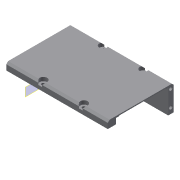
# Autodesk Inventor part: 01_Camera_Module_v0
Saved by Autodesk Inventor 2019 (Build 230136000, 136)
## iProperties
Created: 2021-09-09
Part Number: 01_Camera_Module_v0
Material: Generisch
Document SubType Name: Modeling
Designer: Muriel
Density: 1 g/cm^3
Appearance: Vorgabe
Author: Muriel
Autodesk Inventor part; units mm, degrees
ref_plane "Arbeitsebene6" through (-11.8704, 3.6846, 3.3435) normal (-1, 0, 0) x (0, 1, 0)
sketch "Skizze6" plane through (-11.8704, 3.6846, 3.3435) normal (-1, 0, 0) x (0, 1, 0)
  line L0 (7, 24) -> (7, 1) construction
  line L1 (7, 1) -> (8.5, 1) construction
  line L2 (8.5, 4) -> (8.5, 1) construction
  line L3 (8.5, 4) -> (11.3, 4) construction
  line L4 (11.3, 21) -> (11.3, 4) construction
  line L5 (8.5, 21) -> (11.3, 21) construction
  line L6 (8.5, 24) -> (8.5, 21) construction
  line L7 (7, 24) -> (8.5, 24) construction
  line L8 (8.5, -1) -> (8.5, 1) construction
  line L9 (7, -1) -> (8.5, -1) construction
  line L10 (7, -1) -> (7, 1) construction
  line L11 (8.5, 24) -> (8.5, 26) construction
  line L12 (7, 26) -> (8.5, 26) construction
  line L13 (7, 24) -> (7, 26) construction
  line L14 (12, -6.4) -> (8.1, -6.4)
  line L15 (3.3, 29.4) -> (12, 29.4)
  line L16 (12, 29.4) -> (12, -6.4)
  circle A0 centre (3.1, 20.5) radius 4 construction
  line L17 (7.6, 16) -> (7.6, 25) construction
  line L18 (7.6, 25) -> (-1.4, 25) construction
  line L19 (-1.4, 25) -> (-1.4, 16) construction
  line L20 (-1.4, 16) -> (7.6, 16) construction
  line L21 (3.3, 29.4) -> (-1.9, 29.4)
  line L22 (-1.9, 29.4) -> (-1.9, 11.5)
  line L23 (-1.9, 11.5) -> (8.1, 11.5)
  line L24 (3, 15.9) -> (3, 25.1)
  line L25 (5, 4.25) -> (5, 20.75) projected
  line L26 (11.3, 21) -> (11.3, 4) construction
  line L27 (7.7, 15.9) -> (7.7, 25.1)
  line L28 (7.7, 25.1) -> (-1.5, 25.1)
  line L29 (-1.5, 25.1) -> (-1.5, 15.9)
  line L30 (-1.5, 15.9) -> (7.7, 15.9)
  line L31 (3, 15.9) -> (3, 25.1)
  circle A1 centre (3.1, 20.5) radius 4 construction
  line L32 (7.6, 16) -> (7.6, 25) construction
  line L33 (7.6, 25) -> (-1.4, 25) construction
  line L34 (-1.4, 25) -> (-1.4, 16) construction
  line L35 (-1.4, 16) -> (7.6, 16) construction
  line L36 (-0.7, -1.5) -> (8.3, -1.5) construction
  line L37 (8.5, 7.7) -> (4.1628, 7.7) construction
  line L38 (-0.9, 7.7) -> (-0.9, -1.7) construction
  line L39 (8.1, -6.4) -> (8.1, 3.997) construction
  line L40 (8.1, -6.4) -> (8.1, 11.5)
  line L41 (4.1664, 7.9123) -> (4.1628, 7.7)
  point P0 (3, 11.5)
  dimension "d41" = 13.9
  dimension "d42" = 0.1
  dimension "d48" = 4.3
  dimension "d50" = 9
  dimension "d52" = 17.9
  dimension "d53" = 3.9
  dimension "d54" = 8.9
  dimension "d55" = 17.9
  dimension "d58" = 8.9
  constraints: 36 end point, 4 horizontal, 4 parallel, 4 point on line, 2 perpendicular, 2 vertical, 8 other
  measures "d41" distance between parallel lines of L22 L16
  measures "d42" distance between parallel lines of L20 L30
  measures "d48" distance between parallel lines of L28 L21
  measures "d50" distance from line of L23 A0.centre
  measures "d52" distance between parallel lines of L23 L21
  measures "d53" distance between parallel lines of L16 L40
  measures "d54" distance from line of L21 A1.centre
  measures "d55" distance between parallel lines of L14 L23
  measures "d58" distance from line of L16 A0.centre
ref_plane "Arbeitsebene7" through (-14.9704, 2.9846, -22.1565) normal (-1, 0, 0) x (0, 0, 1)
extrude "Extrusion6" add sketch "Skizze6" along normal up to surface (3.1 mm away)
sketch "Skizze7" plane through (-14.9704, 1.7846, -26.0565) normal (-1, 0, 0) x (0, 0, 1)
  line L0 (4.3, 0.4) -> (13.5, 0.4) projected
  line L1 (4.3, 9.6) -> (4.3, 0.4) projected
  line L2 (13.5, 9.6) -> (4.3, 9.6) projected
  line L3 (13.5, 0.4) -> (13.5, 9.6) projected
  line L4 (35.8, 10) -> (17.9, 10) projected
  line L5 (35.8, 13.9) -> (35.8, 10) projected
  line L6 (0, 13.9) -> (35.8, 13.9) projected
  line L7 (0, 0) -> (0, 13.9) projected
  line L8 (17.9, 0) -> (0, 0) projected
  line L9 (17.9, 10) -> (17.9, 0) projected
  circle A0 centre (8.9, 5) radius 4 construction
  circle A1 centre (8.9, 5) radius 4.2
  point P0 (26.0565, -1.7846)
  dimension "d141" = 8.4
  constraints: 1 centre point, 1 coincident
  measures "d141" diameter of A1
extrude "Extrusion7" add sketch "Skizze7" along normal blind 2 contours L1 L2 L3 L0 | L4 L9 L8 L7 L6 L5
ref_plane "Arbeitsebene8" through (34.8296, 10.6846, -20.6565) normal (1, 0, 0) x (0, 1, 0)
sketch "Skizze8" plane through (-11.8704, 3.6846, 3.3435) normal (1, 0, 0) x (0, 0, -1)
  line L0 (1, 7) -> (24, 7) construction
  line L1 (24, 7) -> (24, 8.5) construction
  line L2 (16.25, 8.5) -> (24, 8.5) construction
  line L3 (8.75, 8.5) -> (16.25, 8.5) construction
  line L4 (1, 8.5) -> (8.75, 8.5) construction
  line L5 (1, 7) -> (1, 8.5) construction
  line L6 (26, 8.5) -> (24, 8.5) construction
  line L7 (26, 7) -> (26, 8.5) construction
  line L8 (26, 7) -> (24, 7) construction
  line L9 (1, 8.5) -> (-1, 8.5) construction
  line L10 (-1, 7) -> (-1, 8.5) construction
  line L11 (1, 7) -> (-1, 7) construction
  line L12 (-6.4, 12) -> (-6.4, 8.1) construction
  line L13 (-6.4, 8.1) -> (11.5, 8.1) construction
  line L14 (11.5, 8.1) -> (11.5, -1.9) construction
  line L15 (11.5, -1.9) -> (29.4, -1.9) construction
  line L16 (29.4, -1.9) -> (29.4, 12) construction
  line L17 (29.4, 12) -> (-6.4, 12) construction
  line L18 (25.1, 7.7) -> (25.1, -1.5) construction
  line L19 (25.1, -1.5) -> (15.9, -1.5) construction
  line L20 (15.9, -1.5) -> (15.9, 7.7) construction
  line L21 (15.9, 7.7) -> (25.1, 7.7) construction
  line L22 (29.4, 12) -> (29.4, -1.9) projected
  line L23 (29.4, 12) -> (-6.4, 12) projected
  line L24 (29.4, -1.9) -> (26.4, -1.9)
  line L25 (26.4, -1.9) -> (26.4, 12)
  line L26 (26.4, 12) -> (29.4, 12)
  line L27 (29.4, 12) -> (29.4, -1.9)
  line L28 (26.4, 12) -> (25.1772, 12)
  line L29 (25.1772, 12) -> (25.1772, 9)
  line L30 (25.1772, 9) -> (26.4, 9)
  line L31 (26.4, 9) -> (26.4, 12)
  line L32 (-6.4, 12) -> (-6.4, 8.1) projected
  line L33 (-6.4, 8.1) -> (11.5, 8.1) projected
  line L34 (-6.4, 12) -> (-2, 12)
  line L35 (-2, 12) -> (-2, 8.1)
  line L36 (-2, 8.1) -> (-6.4, 8.1)
  line L37 (-6.4, 8.1) -> (-6.4, 12)
  line L38 (25.1772, 12) -> (-2, 12)
  line L39 (-2, 12) -> (-2, 12)
  line L40 (25.1772, 11.6) -> (25.1772, 12)
  line L41 (-0.2145, 9) -> (-2, 9)
  line L42 (-2, 9) -> (-2, 12)
  line L43 (-2, 12) -> (-0.2145, 12)
  line L44 (-0.2145, 12) -> (-0.2145, 9)
  line L45 (21, 8.5) -> (4, 8.5) construction
  line L46 (21, 8.5) -> (21, 11.3) construction
  line L47 (4, 11.3) -> (21, 11.3) construction
  line L48 (4, 8.5) -> (4, 11.3) construction
  line L49 (1, 7) -> (-1, 7) construction
  line L50 (29.4, 12) -> (26.4, 12)
  line L51 (26.4, 12) -> (26.4, -1.9)
  line L52 (26.4, -1.9) -> (29.4, -1.9)
  line L53 (29.4, -1.9) -> (29.4, 12)
  line L54 (1, 7) -> (-1, 7) projected
  line L55 (1, 8.5) -> (-1, 8.5) projected
  line L56 (1, 7) -> (24, 7) projected
  line L57 (24, 7) -> (24, 8.5) projected
  line L58 (16.25, 8.5) -> (24, 8.5) projected
  line L59 (8.75, 8.5) -> (16.25, 8.5) projected
  line L60 (1, 8.5) -> (8.75, 8.5) projected
  line L61 (1, 7) -> (1, 8.5) projected
  line L62 (1, 8.5) -> (-1, 8.5) projected
  line L63 (1, 7) -> (-1, 7) projected
  line L64 (1, 7) -> (1, 8.5) projected
  line L65 (-1, 7) -> (-1, 8.5) projected
  line L66 (25.1, -1.5) -> (15.9, -1.5) construction
  line L67 (1, 7) -> (-1, 7) construction
  line L68 (1, 7) -> (-1, 7) construction
  line L69 (-1, 7) -> (-1, 8.5) projected
  line L70 (26.4, -1.9) -> (24.9905, -1.9)
  line L71 (24.9905, -1.9) -> (24.9905, -0.65)
  line L72 (24.9905, -0.65) -> (26.4, -0.65)
  line L73 (26.4, -0.65) -> (26.4, -1.9)
  line L74 (26.4, -0.65) -> (23.4, -0.65)
  line L75 (23.4, -0.65) -> (23.4, 0.1)
  line L76 (23.4, 0.1) -> (26.4, 0.1)
  line L77 (26.4, 0.1) -> (26.4, -0.65)
  line L78 (26.4, 6.5844) -> (25.1772, 6.5844)
  line L79 (25.1772, 6.5844) -> (25.1772, 5.8344)
  line L80 (25.1772, 5.8344) -> (26.4, 5.8344)
  line L81 (26.4, 5.8344) -> (26.4, 6.5844)
  line L82 (-0.2145, 12) -> (25.1772, 12)
  line L83 (25.1772, 12) -> (25.1772, 11.4)
  line L84 (25.1772, 11.4) -> (-0.2145, 11.4)
  line L85 (-0.2145, 11.4) -> (-0.2145, 12)
  point P0 (3.3435, -3.6846)
  point P1 (23, -0.4)
  dimension "d60" = 1
  dimension "d61" = 0.5
  dimension "d63" = 0.5
  dimension "d65" = 0.4
  dimension "d133" = 3
  dimension "d134" = 0.75
  dimension "d135" = 0.75
  dimension "d136" = 0.6
  constraints: 78 end point, 19 parallel, 10 horizontal, 10 perpendicular, 6 point on line, 1 other
  measures "d60" distance between parallel lines of L10 L42
  measures "d61" distance from line of L41 L4.start
  measures "d63" distance between parallel lines of L6 L30
  measures "d65" distance between parallel lines of L25 L7
  measures "d133" distance of L75.end L76.end
  measures "d134" distance of L74.end L75.end
  measures "d135" distance of L79.end L78.end
  measures "d136" distance of L82.end L83.end
extrude "Extrusion8" add sketch "Skizze8" along normal blind 50 contours L22 L24 L25 L23 | L25 L30 L29 L23 | L70 L71 L72 L25 | L29 L84 L44 L23 | L72 L74 L75 L76 L25 | L44 L41 L35 L23 | L25 L80 L79 L78 | L35 L33 L32 L23
sketch "Skizze9" plane through (-16.9704, 15.6846, 9.7435) normal (0, 1, 0) x (1, 0, 0)
  line L0 (55.1, 0) -> (0, 0) projected
  line L1 (0, 35.8) -> (55.1, 35.8) projected
  line L2 (5.1, 7.9) -> (55.1, 7.9) projected
  line L3 (5.1, 3.5) -> (51.8, 3.5)
  line L4 (5.1, 4.4) -> (55.1, 4.4) projected
  line L5 (5.1, 32.8) -> (55.1, 32.8) projected
  line L6 (50.05, 34.05) -> (50.05, 1.75) construction
  line L7 (50.05, 1.75) -> (1.75, 1.75) construction
  line L8 (1.75, 1.75) -> (1.75, 34.05) construction
  line L9 (1.75, 34.05) -> (50.05, 34.05) construction
  line L10 (55.1, 35.8) -> (55.1, 0) projected
  circle A0 centre (40.4228, 1.75) radius 0.9758
  circle A1 centre (18.4228, 1.75) radius 1.1468
  line L11 (0, 0) -> (0, 35.8) projected
  point P0 (16.9704, 9.7435)
  point P1 (51.8, 7.9)
  point P2 (51.8, 3.9)
  point P3 (51.8, 32.3)
  point P4 (7.4228, 34.05)
  point P5 (18.4228, 34.05)
  point P6 (29.4228, 34.05)
  point P7 (40.4228, 34.05)
  point P8 (55.1, 4.4)
  point P9 (55.1, 32.8)
  dimension "d74" = 1.75
  dimension "d75" = 11
  dimension "d76" = 11
  dimension "d77" = 11
  dimension "d140" = 1.75
  constraints: 10 end point, 6 point on line, 2 centre point, 1 horizontal, 4 other
  measures "d74" distance between parallel lines of L1 L9
  measures "d75" distance of point (18.423, 34.05) point (7.423, 34.05)
  measures "d76" distance of point (29.423, 34.05) point (18.423, 34.05)
  measures "d77" distance of point (40.423, 34.05) point (29.423, 34.05)
  measures "d140" distance from line of A1.centre L0
hole "Bohrung1" at (23.4524, 15.6846, -24.3065) at (23.4524, 15.6846, 7.9935) at (1.4524, 15.6846, 7.9935) at (1.4524, 15.6846, -24.3065) direction (0, -1, 0) diameter 1.8 end through all counterbore diameter 4 counterbore depth 2
chamfer "Fase1" distance 1 angle 45 6 edges at (31.2751, 15.6846, -26.0565) (-8.2431, 15.6846, -26.0565) (12.4524, 15.6846, -26.0565) (12.4524, 15.6846, 9.7435) (-8.2431, 15.6846, 9.7435) (31.2751, 15.6846, 9.7435)
chamfer "Fase2" distance 1 angle 45 1 edges at (-11.8704, 6.7846, -12.5565)
sketch "Skizze11" plane through (34.8296, 1.9846, -26.0565) normal (0, 0, -1) x (-1, 0, 0)
  line L0 (49.8, 0.2) -> (49.8, 9.4) projected
  line L1 (47.7, 0.2) -> (47.7, 9.4) projected
  circle A0 centre (47.7, 4.8) radius 1.4
  point P0 (34.8296, -1.9846)
  dimension "d93" = 2.8
  constraints: 1 centre point, 1 midpoint
  measures "d93" diameter of A0
extrude "Extrusion10" cut sketch "Skizze11" against normal blind 10
sketch "Skizze12" plane through (-16.9704, 1.7846, -8.1565) normal (0, -1, 0) x (1, 0, 0)
  line L0 (5.1, -12.9) -> (55.1, -12.9) projected
  line L1 (5.1, -14.9) -> (55.1, -14.9) projected
  line L2 (5.1, -12.9) -> (55.1, -12.9) projected
  line L3 (5.1, -14.9) -> (5.1, -13.6) projected
  line L4 (5.1, -14.9) -> (55.1, -14.9) projected
  line L5 (55.1, -12.9) -> (55.1, -14.9) projected
  line L6 (55.1, -14.9) -> (41.1, -14.9)
  line L7 (41.1, -14.9) -> (41.1, -8.3617)
  line L8 (41.1, -8.3617) -> (55.1, -8.3617)
  line L9 (55.1, -8.3617) -> (55.1, -14.9)
  line L10 (5.1, -13.6772) -> (55.1, -13.6772) projected
  line L11 (5.1, -25.06) -> (5.1, 25.06) projected
  line L12 (5.1, -14.9) -> (21.1, -14.9)
  line L13 (21.1, -14.9) -> (21.1, -8.3617)
  line L14 (21.1, -8.3617) -> (5.1, -8.3617)
  line L15 (5.1, -8.3617) -> (5.1, -14.9)
  line L16 (5.1, -12.9) -> (5.1, -13.6) projected
  point P0 (16.9704, 8.1565)
  point P1 (51.8, -13.4)
  point P2 (51.8, -14.4)
  point P3 (5.1, -13.9)
  point P4 (5.1, -13.9)
  dimension "d113" = 36
  dimension "d132" = 0
  constraints: 16 end point, 4 parallel, 2 horizontal, 2 perpendicular, 1 point on line, 2 other
  measures "d113" distance between parallel lines of L7 L11
  measures "d132" distance from line of point (5.1, -14.9) L15
ref_plane "Arbeitsebene9" through (-11.8704, 12.1846, -22.6565) normal (0, 1, 0) x (0, 0, 1)
extrude "Extrusion11" cut sketch "Skizze12" against normal blind 13 contours L11 L14 L13 L0 | L0 L13 L10 L3 L11 | L7 L8 L9 L0 | L0 L5 L10 L7 | L13 L1 L3 L10 | L10 L5 L1 L7
sketch "Skizze13" plane through (38.1296, 10.1846, -23.0565) normal (1, 0, 0) x (0, 0, -1)
  line L0 (-32.3, 4.7) -> (-31.3, 5.7) projected
  line L1 (-32.3, 1.8) -> (-32.3, 4.7) projected
  line L2 (-28.4, 1.8) -> (-32.3, 1.8) projected
  line L3 (-28.4, 2.2) -> (-28.4, 1.8) projected
  line L4 (-24.4, 2.2) -> (-28.4, 2.2) projected
  line L5 (-24.4, 4.1) -> (-24.4, 2.2) projected
  line L6 (-4, 5.1) -> (-23.4, 5.1) projected
  line L7 (-3, 2.5) -> (-3, 4.1) projected
  line L8 (0, 2.5) -> (-3, 2.5) projected
  line L9 (0, 0) -> (0, 2.5) projected
  line L10 (-1, 0) -> (0, 0) projected
  line L11 (-1, -2) -> (-1, 0) projected
  line L12 (0, -4.4) -> (0, -3) projected
  line L13 (-1, -6.4) -> (-1, -5.4) projected
  line L14 (0, -6.4) -> (-1, -6.4) projected
  line L15 (0, -8.2) -> (0, -6.4) projected
  line L16 (3.5, -8.2) -> (0, -8.2) projected
  line L17 (3.5, 4.7) -> (3.5, -8.2) projected
  line L18 (2.5, 5.7) -> (3.5, 4.7) projected
  line L19 (-31.3, 5.7) -> (2.5, 5.7) projected
  circle A0 centre (1.4, -5.4) radius 0.9
  circle A1 centre (1.4, 3.4) radius 0.9
  line L20 (-23.4, 5.1) -> (-24.4, 4.1) projected
  line L21 (-3, 4.1) -> (-4, 5.1) projected
  line L22 (0, -3) -> (-1, -2) projected
  line L23 (-1, -5.4) -> (0, -4.4) projected
  point P0 (-23.0565, -10.1846)
  dimension "d101" = 1.8
  dimension "d102" = 1.8
  constraints: 2 centre point
  measures "d101" diameter of A0
  measures "d102" diameter of A1
extrude "Extrusion12" cut sketch "Skizze13" against normal blind 8 contours A0 | A1
sketch "Skizze15" plane through (-16.9704, 11.7846, -8.1565) normal (0, -1, 0) x (1, 0, 0)
  line L0 (5.1, 0) -> (0, 0) projected
  line L1 (5.1, 13.5) -> (5.1, 0) projected
  line L2 (0, 17.9) -> (55.1, 17.9) projected
  line L3 (13.1, 13.5131) -> (21.1, 13.5131)
  line L4 (21.1, 13.5131) -> (21.1, 8.0131)
  line L5 (21.1, 8.0131) -> (13.1, 8.0131)
  line L6 (13.1, 8.0131) -> (13.1, 13.5131)
  line L7 (41.1, -14.9) -> (41.1, -13.6772) projected
  line L8 (5.1, 13.5) -> (55.1, 13.5) projected
  line L9 (55.1, 84.35) -> (55.1, 11.7145) projected
  line L10 (41.1, 13.5) -> (55.1, 13.5)
  line L11 (55.1, 13.5) -> (55.1, 8)
  line L12 (55.1, 8) -> (41.1, 8)
  line L13 (41.1, 8) -> (41.1, 13.5)
  line L14 (41.1, -14.9) -> (55.1, -14.9)
  line L15 (55.1, -14.9) -> (55.1, -9.4)
  line L16 (55.1, -9.4) -> (41.1, -9.4)
  line L17 (41.1, -9.4) -> (41.1, -14.9)
  line L18 (5.1, 13.5) -> (55.1, 13.5) projected
  line L19 (55.1, 17.9) -> (55.1, 13.5) projected
  line L20 (0, 0) -> (0, 17.9) projected
  point P0 (16.9704, 8.1565)
  point P1 (134.9, 84.35)
  dimension "d116" = 8
  dimension "d117" = 8
  dimension "d120" = 5.5
  dimension "d122" = 5.5
  constraints: 24 end point, 6 parallel, 3 horizontal, 3 perpendicular, 2 point on line, 2 other
  measures "d116" distance of L4.end L5.end
  measures "d117" distance between parallel lines of L6 L1
  measures "d120" distance between parallel lines of L5 L3
  measures "d122" distance between parallel lines of L14 L16
extrude "Extrusion14" cut sketch "Skizze15" against normal blind 3 contours L8 L4 L5 L6 | L6 L3 L4 L8 | L9 L11 L12 L13 L8 | L7 L17 L16 L15 L14
chamfer "Fase4" distance 3 angle 45 1 edges at (-11.8704, 11.3846, -16.6565)
ref_plane "Arbeitsebene10" through (30.8296, 14.9846, -11.9065) normal (0, 1, 0) x (0, 0, 1)
chamfer "Fase5" distance 1 angle 45 5 edges at (14.1296, 3.7846, -23.0565) (14.1296, 3.0346, -21.647) (14.1296, 9.519, -23.0565) (14.1296, 10.269, -23.0565) (14.1296, 12.6846, -23.0565)
